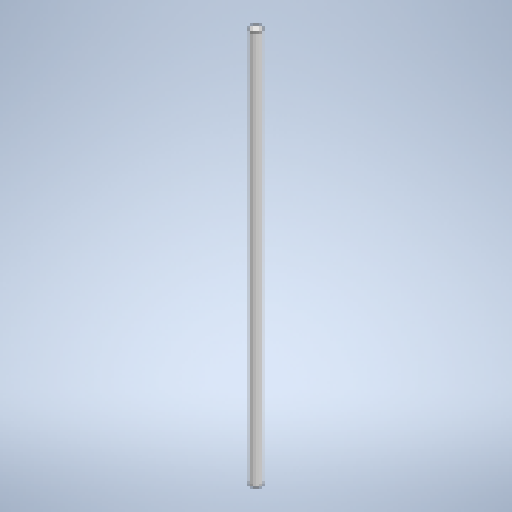
# Autodesk Inventor part: пруток
Saved by Autodesk Inventor 2025 (Build 290162010, 162A)
## iProperties
Created: 2024-09-17
Part Number: пруток
Material: Generic
Document SubType Name: Modeling
Designer: pokla
Density: 1 g/cm^3
Appearance: Default
Author: pokla
Autodesk Inventor part; units mm, degrees
ref_plane "YZ Plane" through (0, 0, 0) normal (1, 0, 0) x (0, 1, 0)
ref_plane "XZ Plane" through (0, 0, 0) normal (0, 1, 0) x (-1, 0, 0)
ref_plane "XY Plane" through (0, 0, 0) normal (0, 0, 1) x (1, 0, 0)
sketch "Sketch1" plane through (0, 0, 0) normal (0, 0, 1) x (1, 0, 0)
  circle A0 centre (0, 0) radius 9
  dimension "d0" = 18
  constraints: 1 centre point, 1 coincident
  measures "d0" diameter of A0
extrude "Extrusion1" add sketch "Sketch1" along normal blind 720
body "Solid1"
